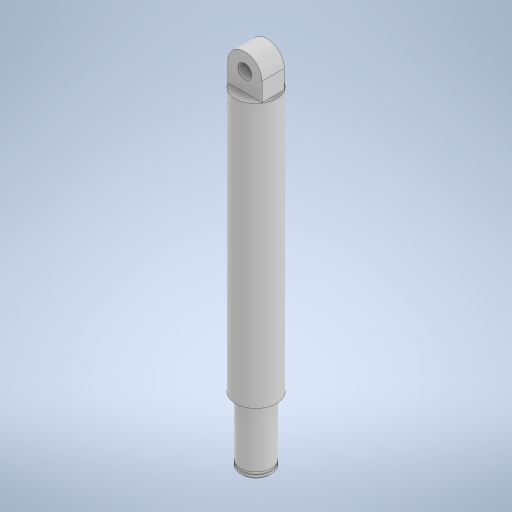
# Autodesk Inventor part: 14_Eje
Saved by Autodesk Inventor 2024.2 (Build 282272000, 272)
## iProperties
Created: 2024-04-27
Part Number: 14_Eje
Material: Genérico
Document SubType Name: Modeling
Designer: Cosmic Dinodog
Density: 1 g/cm^3
Appearance: Valor por defecto
Author: Cosmic Dinodog
Autodesk Inventor part; units mm, degrees
ref_plane "YZ Plane" through (0, 0, 0) normal (1, 0, 0) x (0, 1, 0)
ref_plane "XZ Plane" through (0, 0, 0) normal (0, 1, 0) x (-1, 0, 0)
ref_plane "XY Plane" through (0, 0, 0) normal (0, 0, 1) x (1, 0, 0)
sketch "Boceto1" plane through (0, 0, 0) normal (0, 1, 0) x (-1, 0, 0)
  circle A0 centre (0, 0) radius 9
  dimension "d0" = 18
  constraints: 1 centre point, 1 coincident
  measures "d0" diameter of A0
extrude "Extrusión1" add sketch "Boceto1" along normal blind 38
sketch "Boceto2" plane through (0, 38, 0) normal (0, 1, 0) x (1, 0, 0)
  circle A0 centre (0, 0) radius 12
  dimension "d3" = 24
  constraints: 1 centre point, 1 coincident
  measures "d3" diameter of A0
extrude "Extrusión2" add sketch "Boceto2" along normal blind 154
sketch "Boceto3" plane through (0, 0, 0) normal (0, 0, 1) x (1, 0, 0)
  line L0 (0, 0) -> (0, 203) construction
  circle A0 centre (0, 203) radius 4
  arc A1 (10, 203) -> (-10, 203) centre (0, 203) ccw
  line L1 (10, 203) -> (10, 192)
  line L2 (12, 192) -> (-12, 192) projected
  line L3 (-10, 192) -> (-10, 203)
  line L4 (-10, 192) -> (10, 192)
  dimension "d6" = 203
  dimension "d7" = 8
  dimension "d8" = 20
  dimension "d9" = 20
  constraints: 8 end point, 2 centre point, 2 coincident, 2 point on circle, 2 point on line, 2 vertical, 1 collinear, 1 tangent
  measures "d6" distance of L0.start L0.end
  measures "d7" diameter of A0
  measures "d8" diameter of A1
  measures "d9" distance between parallel lines of L1 L3
extrude "Extrusión3" add sketch "Boceto3" along normal mid plane 13
sketch "Boceto4" plane through (0, 0, 0) normal (0, 0, 1) x (1, 0, 0)
  line L0 (0, 0) -> (0, 3.8) construction
  line L1 (0, 3.8) -> (9, 3.8) construction
  line L2 (9, 0) -> (9, 38) projected
  line L3 (9, 3.8) -> (9, 2.3)
  line L4 (9, 2.3) -> (8.5, 2.3)
  line L5 (8.5, 2.3) -> (8.5, 3.8)
  line L6 (8.5, 3.8) -> (9, 3.8)
  dimension "d12" = 3.8
  dimension "d13" = 1.5
  dimension "d14" = 0.5
  constraints: 12 end point, 3 point on line, 1 collinear, 1 horizontal, 1 parallel, 1 perpendicular, 1 vertical
  measures "d12" distance of L0.start L0.end
  measures "d13" distance of L1.end L3.end
  measures "d14" distance of L3.end L4.end
revolve "Revolución1" cut sketch "Boceto4" angle 360 about axis through (0, 0, 0) along (0, 1, 0)
chamfer "Chaflán1" distance 1 angle 45 1 edges at (9, 0, 0) measured on face at (-2.2455, 0, -1.9894)
